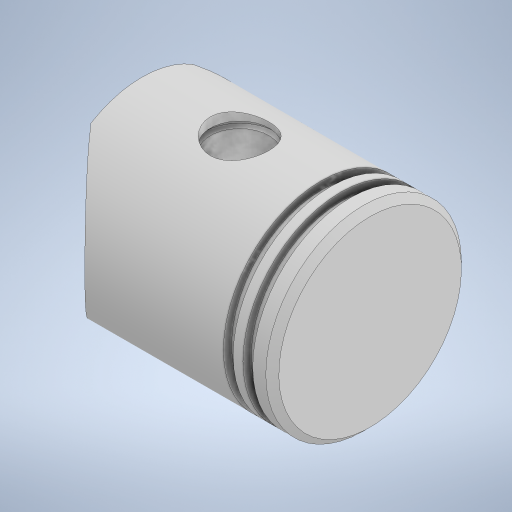
# Autodesk Inventor part: 02
Saved by Autodesk Inventor 2023 (Build 270158000, 158)
## iProperties
Created: 2023-09-22
Part Number: 02
Material: Genérico
Document SubType Name: Modeling
Designer: User
Density: 1 g/cm^3
Appearance: Padrão
Author: User
Autodesk Inventor part; units mm, degrees
ref_plane "YZ Plane" through (0, 0, 0) normal (1, 0, 0) x (0, 1, 0)
ref_plane "XZ Plane" through (0, 0, 0) normal (0, 1, 0) x (-1, 0, 0)
ref_plane "XY Plane" through (0, 0, 0) normal (0, 0, 1) x (1, 0, 0)
sketch "Esboço1" plane through (0, 0, 0) normal (0, 0, 1) x (1, 0, 0)
  line L0 (0, 0) -> (-70, 0)
  line L1 (0, 0) -> (0, 30)
  line L2 (-70, 30) -> (-70, 28)
  line L3 (-70, 28) -> (-18, 28)
  line L4 (-18, 28) -> (-58.0179, 28)
  line L5 (-18, 28) -> (-18, 25)
  line L6 (-18, 25) -> (-6, 25)
  line L7 (-6, 25) -> (-6, 0)
  line L8 (0, 30) -> (-6, 30)
  line L9 (-6, 30) -> (-6, 27.5)
  line L10 (-6, 27.5) -> (-9, 27.5)
  line L11 (-9, 27.5) -> (-9, 30)
  line L12 (-9, 30) -> (-12, 30)
  line L13 (-12, 30) -> (-12, 27.5)
  line L14 (-12, 27.5) -> (-15, 27.5)
  line L15 (-15, 27.5) -> (-15, 30)
  line L16 (-15, 30) -> (-70, 30)
  line L17 (-6, 0) -> (0, 0)
  dimension "d1" = 60
  dimension "d2" = 70
  dimension "d4" = 70
  dimension "d5" = 56
  dimension "d8" = 52
  dimension "d9" = 64
  dimension "d10" = 50
  dimension "d11" = 6
  dimension "d12" = 55
  dimension "d13" = 3
  dimension "d14" = 3
  dimension "d15" = 3
  dimension "d16" = 55
  dimension "d17" = 55
  dimension "d18" = 60
  constraints: 36 end point, 6 perpendicular, 5 horizontal, 5 vertical, 2 point on line, 1 collinear
  measures "d1" diameter of L1.end L0
  measures "d2" distance of L0.start L0.end
  measures "d4" distance of L1.end L2.start
  measures "d5" diameter of L2.end L0
  measures "d8" distance of L2.end L3.end
  measures "d9" distance from line of L6.end L2
  measures "d10" diameter of L6 L0
  measures "d11" distance of L1.end L8.end
  measures "d12" diameter of L9.end L0
  measures "d13" distance between parallel lines of L9 L11
  measures "d14" distance between parallel lines of L11 L13
  measures "d15" distance between parallel lines of L13 L15
  measures "d16" diameter of L14 L0
  measures "d17" distance of L15.end L2.start
  measures "d18" diameter of L12 L0
revolve "Revolução1" add sketch "Esboço1" angle 360 about axis through (0, 0, 0) along (-1, 0, 0)
chamfer "Chanfro1" distance 2 angle 45 1 edges at (0, -30, 0)
fillet "Arredondamento1" radius 2 1 edges at (-18, -28, 0)
sketch "Esboço2" plane through (0, 0, 0) normal (0, 0, 1) x (1, 0, 0)
  line L0 (-70, 0) -> (-40, 0)
  line L1 (-70, 0) -> (-90, 0)
  circle A0 centre (-90, 0) radius 32.5
  point P0 (0, 0)
  dimension "d24" = 70
  dimension "d25" = 30
  dimension "d26" = 20
  dimension "d27" = 65
  dimension "d28" = 90
  constraints: 4 end point, 1 centre point, 1 coincident, 1 horizontal
  measures "d24" distance of point (0, 0) L0.start
  measures "d25" distance of L0.start L0.end
  measures "d26" distance of L0.start L1.end
  measures "d27" diameter of A0
  measures "d28" distance of point (0, 0) L1.end
extrude "Extrusão1" cut sketch "Esboço2" along normal mid plane 200000
sketch "Esboço3" plane through (0, 0, 0) normal (0, 1, 0) x (-1, 0, 0)
  line L0 (70, -15.6125) -> (70, 15.6125) projected
  line L1 (70, 0) -> (40, 0)
  line L2 (70, -15.6125) -> (70, 15.6125) projected
  circle A0 centre (40, 0) radius 12.5
  point P0 (0, 0)
  dimension "d32" = 30
  dimension "d33" = 25
  constraints: 2 end point, 2 midpoint, 1 centre point, 1 coincident, 1 horizontal
  measures "d32" distance of L1.end point (70, 0)
  measures "d33" diameter of A0
extrude "Extrusão2" add sketch "Esboço3" along normal up to next
sketch "Esboço4" plane through (-40, 0, 0) normal (0, -1, 0) x (1, 0, 0)
  circle A0 centre (0, 0) radius 12.5
  point P0 (40, 0)
  constraints: 1 centre point
extrude "Extrusão3" add sketch "Esboço4" along normal up to next
sketch "Esboço5" plane through (-6, 0, 0) normal (-1, 0, 0) x (0, 0, 1)
  line L0 (-17.5, -10) -> (17.5, -10)
  line L1 (17.5, -10) -> (17.5, 10)
  line L2 (17.5, 10) -> (-17.5, 10)
  line L3 (-17.5, 10) -> (-17.5, -10)
  line L4 (-17.5, -10) -> (17.5, 10) construction
  line L5 (17.5, -10) -> (-17.5, 10) construction
  point P0 (0, 0)
  dimension "d38" = 20
  constraints: 12 end point, 2 midpoint, 2 parallel, 1 horizontal, 1 perpendicular
  measures "d38" distance between parallel lines of L0 L2
extrude "Extrusão4" cut sketch "Esboço5" along normal blind 100
sketch "Esboço6" plane through (-40, 10, 0) normal (0, -1, 0) x (1, 0, 0)
  circle A0 centre (0, 0) radius 12.5 projected
  circle A1 centre (0, 0) radius 9
  point P0 (40, 0)
  dimension "d41" = 18
  constraints: 1 centre point, 1 coincident
  measures "d41" diameter of A1
extrude "Extrusão5" cut sketch "Esboço6" along normal mid plane 100 contours A1
sketch "Esboço8" plane through (0, 0, 0) normal (0, 0, 1) x (1, 0, 0)
  line L0 (0, 0) -> (-31, 0)
  line L1 (-31, 27) -> (-29, 27)
  line L2 (-29, 27) -> (-29, 25)
  line L3 (-29, 25) -> (-31, 25)
  line L4 (-31, 27) -> (-31, 25)
  line L5 (-31, -27) -> (-29, -27)
  line L6 (-29, -27) -> (-29, -25)
  line L7 (-29, -25) -> (-31, -25)
  line L8 (-31, -27) -> (-31, -25)
  line L9 (-49, 30) -> (-49, 10) projected
  line L10 (-40, 30) -> (-40, -34.5055)
  point P0 (-31, 30)
  dimension "d45" = 3
  dimension "d46" = 2
  dimension "d47" = 2
  dimension "d49" = 18
  constraints: 20 end point, 4 symmetric about line, 2 horizontal, 1 perpendicular, 1 vertical
  measures "d45" distance of point (-31, 30) L1.start
  measures "d46" distance of L1.start L1.end
  measures "d47" distance of L1.end L2.end
  measures "d49" diameter of L9 L10
revolve "Revolução2" cut sketch "Esboço8" angle 360 about axis through (-40, 30, 0) along (0, -1, 0)
